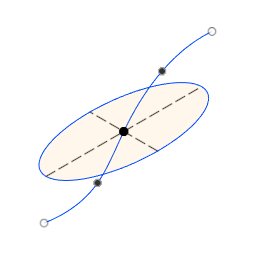
7.4 intersection  curve (Autodesk Fusion 360 design; units mm, degrees)
Autodesk Fusion 360 part; units mm, degrees
sketch "Sketch1" plane through (0, 0, 0) normal (0, 0, 1) x (1, 0, 0)
  ellipse E0 centre (0, 0) end of major axis (0, 44.4558) minor radius 19.3308
  line L0 (0, -44.4558) -> (0, 44.4558)
  line L1 (19.3308, 0) -> (-19.3308, 0)
  constraint coincident E0.centre origin
  constraint vertical L0
  constraint coincident E0 L0.start
  constraint coincident E0 L0.end
  constraint coincident E0 L1.start
  constraint coincident E0 L1.end
sketch "Sketch2" plane through (0, 0, 0) normal (1, 0, 0) x (0, 1, 0)
  spline S0 degree 5 poles (-45.5975, -22.5304) (-44.017, -22.7708) (-40.9362, -23.1724) (-36.5554, -23.5372) (-31.1971, -23.5463) (-25.3047, -22.7575) (-20.2, -21.1746) (-15.8307, -18.8258) (-12.0952, -15.7728) (-8.8194, -12.1268) (-5.7807, -8.0388) (-2.7469, -3.6809) (0.4907, 0.7685) (4.0788, 5.1411) (8.075, 9.2917) (12.4751, 13.097) (17.2341, 16.4558) (22.2874, 19.2902) (27.5718, 21.5469) (33.0444, 23.1989) (38.6781, 24.2368) (43.302, 24.577) (46.8328, 24.5589) (49.2146, 24.4258) (50.4125, 24.3291) knots 0 0 0 0 0 0 0.05 0.1 0.15 0.2 0.25 0.3 0.35 0.4 0.45 0.5 0.55 0.6 0.65 0.7 0.75 0.8 0.85 0.9 0.95 1 1 1 1 1 1
  point P0 (-14.9826, -17.9486)
  point P1 (21.8803, 18.9142)
sketch "Sketch4" plane through (0, 0, 0) normal (1, 0, 0) x (0, 1, 0)
  circle A0 centre (0, 0) radius 19.7423
  constraint coincident A0.centre origin
extrude "Extrude1" add sketch "Sketch4" along normal mid plane 57.758
hidden bodies 1
